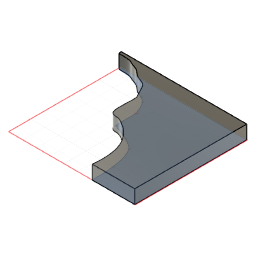
Jack mod v3 (Autodesk Fusion 360 design; units mm, degrees)
Autodesk Fusion 360 part; units mm, degrees
sketch "Sketch3" plane through (0, 0, 0) normal (0, 0, 1) x (1, 0, 0)
  spline S0 degree 5 poles (-22.7464, 19.4495) (-22.469, 19.4525) (-21.9349, 19.455) (-21.1958, 19.4489) (-20.3347, 19.4209) (-19.4632, 19.353) (-18.7871, 19.2537) (-18.2855, 19.1264) (-17.9222, 18.9768) (-17.6402, 18.8139) (-17.361, 18.6501) (-17.0122, 18.4933) (-16.5515, 18.3403) (-15.9914, 18.1709) (-15.3759, 17.9575) (-14.7589, 17.6759) (-14.1845, 17.3143) (-13.6608, 16.8861) (-13.1595, 16.4272) (-12.6377, 15.9809) (-12.0542, 15.585) (-11.3859, 15.2599) (-10.6502, 14.9915) (-9.9012, 14.7344) (-9.2049, 14.4312) (-8.6129, 14.0321) (-8.1504, 13.5055) (-7.7658, 12.8743) (-7.401, 12.1698) (-7.0256, 11.4075) (-6.6186, 10.599) (-6.2604, 9.9194) (-5.9719, 9.3923) (-5.7708, 9.033) (-5.668, 8.8515) knots 0 0 0 0 0 0 0.033333 0.066667 0.1 0.133333 0.166667 0.2 0.233333 0.266667 0.3 0.333333 0.366667 0.4 0.433333 0.466667 0.5 0.533333 0.566667 0.6 0.633333 0.666667 0.7 0.733333 0.766667 0.8 0.833333 0.866667 0.9 0.933333 0.966667 1 1 1 1 1 1
  line L0 (-9.4823, 15.1452) -> (-7, 12)
  spline S1 degree 5 poles (-5.668, 8.8515) (-5.6566, 8.7435) (-5.6363, 8.5169) (-5.6136, 8.1447) (-5.599, 7.5838) (-5.6057, 6.7757) (-5.6339, 5.8662) (-5.6757, 4.8686) (-5.7179, 3.8075) (-5.7396, 2.7215) (-5.7131, 1.6608) (-5.6035, 0.6863) (-5.3684, -0.1323) (-4.9579, -0.7173) (-4.3119, -0.9817) (-3.4956, -1.0494) (-2.6134, -1.0998) (-1.7744, -1.3059) (-1.019, -1.6914) (-0.3088, -2.1288) (0.3628, -2.5797) (0.8769, -2.9251) (1.2499, -3.1731) (1.4931, -3.3333) (1.6133, -3.4121) knots 0 0 0 0 0 0 0.05 0.1 0.15 0.2 0.25 0.3 0.35 0.4 0.45 0.5 0.55 0.6 0.65 0.7 0.75 0.8 0.85 0.9 0.95 1 1 1 1 1 1
  line L1 (-6.3206, 1.2823) -> (-4, -2)
  line L2 (-4.3259, -0.3256) -> (1.0054, -2.4768)
  spline S2 degree 5 poles (1.6133, -3.4121) (1.8952, -3.6327) (2.4442, -4.0849) (3.2232, -4.796) (4.1714, -5.8109) (5.1959, -7.198) (6.0468, -8.7131) (6.7125, -10.3649) (7.1909, -12.1548) (7.4937, -14.0742) (7.6361, -16.1119) (7.6332, -17.8283) (7.5696, -19.1609) (7.5003, -20.0691) (7.459, -20.5281) knots 0 0 0 0 0 0 0.1 0.2 0.3 0.4 0.5 0.6 0.7 0.8 0.9 1 1 1 1 1 1
  line L3 (7.459, -20.5281) -> (23, -20.5281)
  line L4 (23, -20.5281) -> (23, 20.4719)
  line L5 (23, 20.4719) -> (-23, 20.4719)
  line L6 (-23, 20.4719) -> (-22.7464, 19.4495)
  point P0 (-18, 19)
  point P1 (-17, 18.5)
  point P2 (-14.5, 17.5)
  point P3 (-11.7093, 15.4298)
  point P4 (-8.2411, 13.5726)
  point P5 (-5.668, 5.0477)
  point P6 (-5.1603, -0.3588)
  point P7 (-1.6602, -1.4012)
  point P8 (6.4769, -9.8657)
  dimension "d1" = 41
  constraint midpoint P4 L0
  constraint midpoint P6 L1
  constraint midpoint P7 L2
  constraint horizontal L3
  constraint perpendicular L3 L4
  constraint perpendicular L4 L5
  measures "d1" distance of L3.end L4.end
extrude "Extrude1" add sketch "Sketch3" along normal blind 5
